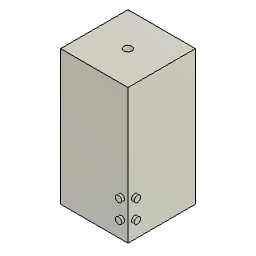
Step2-LegExtension-4X (Autodesk Fusion 360 design; units mm, degrees)
Autodesk Fusion 360 part; units mm, degrees
note: some values were not read from the file. Set by a fixed rule: which sketch regions a step uses.
sketch "Sketch1" plane through (0, 0, 0) normal (0, 0, 1) x (1, 0, 0)
  line L0 (0, 0) -> (-50, 0)
  line L1 (-50, 0) -> (-50, 50)
  line L2 (-50, 50) -> (0, 50)
  line L3 (0, 50) -> (0, 0)
  dimension "d1" = 50
  dimension "d2" = 50
  constraint horizontal L0
  constraint vertical L1
  constraint horizontal L2
  constraint vertical L3
  constraint coincident L0.start L3.end
  measures "d1" distance of L0.start L0.end
  measures "d2" distance of L0.start L2.end
extrude "Extrude1" add sketch "Sketch1" along normal blind 100
ref_plane "WorkPlane1" through (-25, 25, 0) normal (0, 0, -1) x (-1, 0, 0)
sketch "Sketch2" plane through (-25, 25, 0) normal (0, 0, -1) x (1, 0, 0)
  circle A0 centre (0, 0) radius 12.5
  dimension "d6" = 25
  constraint coincident A0.centre origin
  measures "d6" diameter of A0
extrude "Extrude2" cut sketch "Sketch2" against normal blind 50 draft -20
sketch "Sketch3" plane through (0, 0, 0) normal (0, 0, -1) x (1, 0, 0)
  circle A0 centre (-25, -25) radius 12.5
  line L0 (-50, -50) -> (0, -50)
  line L1 (0, -50) -> (0, 0)
  line L2 (0, 0) -> (-50, 0)
  line L3 (-50, 0) -> (-50, -50)
ref_plane "WorkPlane2" through (-25, 25, 0) normal (0, 0, -1) x (1, 0, 0)
sketch "Sketch4" plane through (0, 0, 0) normal (0, 0, -1) x (1, 0, 0)
  circle A0 centre (-25, -25) radius 3
  circle A1 centre (-25, -25) radius 4.75
  dimension "d10" = 6
  dimension "d11" = 9.5
  constraint concentric A0 A1
  measures "d10" diameter of A0
  measures "d11" diameter of A1
extrude "Extrude3" cut sketch "Sketch4" against normal blind 100 contours A0
sketch "Sketch5" plane through (-25, 25, 0) normal (0, 0, -1) x (1, 0, 0)
  circle A0 centre (0, 0) radius 4.75
  dimension "d14" = 9.5
  constraint coincident A0.centre origin
  measures "d14" diameter of A0
extrude "Extrude4" cut sketch "Sketch5" against normal blind 80
sketch "Sketch6" plane through (0, 0, 0) normal (0, 0, -1) x (1, 0, 0)
ref_plane "WorkPlane3" through (0, 25, 50) normal (1, 0, 0) x (0, 1, 0)
sketch "Sketch7" plane through (0, 25, 50) normal (1, 0, 0) x (0, 1, 0)
  line L0 (-25, -50) -> (-20, -50)
  line L1 (-20, -50) -> (-20, -37)
  line L2 (-20, -37) -> (-25, -37)
  line L3 (-25, -37) -> (-25, -50)
  line L4 (-25, -37) -> (-20, -37)
  line L5 (-20, -37) -> (-20, -23)
  line L6 (-20, -23) -> (-25, -23)
  line L7 (-25, -23) -> (-25, -37)
  circle A0 centre (-20, -23) radius 2.4
  circle A1 centre (-20, -37) radius 2.4
  dimension "d18" = 5
  dimension "d19" = 13
  dimension "d20" = 5
  dimension "d21" = 14
  dimension "d22" = 4.8
  dimension "d23" = 4.8
  constraint horizontal L0
  constraint vertical L1
  constraint horizontal L2
  constraint vertical L3
  constraint horizontal L4
  constraint vertical L5
  constraint horizontal L6
  constraint vertical L7
  constraint coincident L5.end L6.start
  constraint coincident L1.end L2.start
  measures "d18" distance of L0.start L0.end
  measures "d19" distance of L0.start L2.end
  measures "d20" distance of L2.end L1.end
  measures "d21" distance of L2.end L6.end
  measures "d22" diameter of A0
  measures "d23" diameter of A1
extrude "Extrude5" add sketch "Sketch7" along normal blind 2 contours L1 L2 L4 A1 | L1 L5 A1 | L2 L4 L5 A1 | L5 L6 A0 | L5 L6 A0
ref_plane "WorkPlane4" through (-25, 0, 50) normal (0, -1, 0) x (1, 0, 0)
sketch "Sketch8" plane through (-25, 0, 50) normal (0, -1, 0) x (1, 0, 0)
  line L0 (25, -50) -> (20, -50)
  line L1 (20, -50) -> (20, -37)
  line L2 (20, -37) -> (25, -37)
  line L3 (25, -37) -> (25, -50)
  line L4 (25, -37) -> (20, -37)
  line L5 (20, -37) -> (20, -23)
  line L6 (20, -23) -> (25, -23)
  line L7 (25, -23) -> (25, -37)
  circle A0 centre (20, -23) radius 2.4
  circle A1 centre (20, -37) radius 2.4
  dimension "d27" = 4.8
  dimension "d28" = 4.8
  constraint horizontal L0
  constraint vertical L1
  constraint horizontal L2
  constraint vertical L3
  constraint horizontal L4
  constraint vertical L5
  constraint horizontal L6
  constraint vertical L7
  constraint coincident L5.end L6.start
  constraint coincident L1.end L2.start
  measures "d27" diameter of A0
  measures "d28" diameter of A1
extrude "Extrude6" add sketch "Sketch8" along normal blind 2 contours L1 L5 A1 | L1 L2 L4 A1 | L2 L4 L5 A1 | L5 L6 A0 | L5 L6 A0
